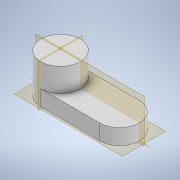
# Autodesk Inventor part: Roof_Pin_Clip
Saved by Autodesk Inventor 2022.4 (Build 264492010, 492A)
## iProperties
Created: 2025-04-04
Part Number: Roof_Pin_Clip
Material: Generic
Document SubType Name: Modeling
Designer: jan-m
Density: 1 g/cm^3
Appearance: Default
Author: jan-m
Autodesk Inventor part; units mm, degrees
sketch "Sketch1" plane through (0, 0, 0) normal (0, 1, 0) x (-1, 0, 0)
  circle A0 centre (0, 0) radius 2.5
  line L0 (0, -2.5) -> (-7.5, -2.5)
  line L1 (-7.5, -2.5) -> (-7.5, 2.5)
  line L2 (-7.5, 2.5) -> (0, 2.5)
  circle A1 centre (-7.5, 0) radius 2.5
  line L3 (-12.325, 0) -> (4.825, 0) projected
  point P0 (-7.5, 2.5)
  point P1 (2.5, 0)
  dimension "d14" = 5
  dimension "d0" = 5
  dimension "d1" = 7.5
  dimension "d13" = 7.5
  constraints: 6 end point, 3 point on circle, 2 tangent, 1 centre point, 1 coincident, 1 horizontal, 1 midpoint, 1 perpendicular, 1 point on line, 3 other
  measures "d0" diameter of A0
  measures "d1" distance of L0.start L0.end
  measures "d13" distance of L1.end L2.end
extrude "Extrusion1" add sketch "Sketch1" along normal blind 5 contours L3 A0 | A0 L3
extrude "Extrusion2" add sketch "Sketch1" along normal blind 2
body "Solid1"
